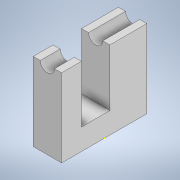
# Autodesk Inventor part: shaft_support
Saved by Autodesk Inventor 2021 (Build 250183000, 183)
## iProperties
Created: 2021-04-13
Part Number: shaft_support
Material: Generic
Document SubType Name: Modeling
Designer: Jawal
Density: 1 g/cm^3
Appearance: Default
Author: Jawal
Autodesk Inventor part; units mm, degrees
note: some values were not read from the file. Chosen so that the rebuilt part matches the saved one: direction of "Emboss1".
ref_plane "YZ Plane" through (0, 0, 0) normal (1, 0, 0) x (0, 1, 0)
ref_plane "XZ Plane" through (0, 0, 0) normal (0, 1, 0) x (-1, 0, 0)
ref_plane "XY Plane" through (0, 0, 0) normal (0, 0, 1) x (1, 0, 0)
sketch "Sketch1" plane through (0, 0, 0) normal (0, 1, 0) x (-1, 0, 0)
  line L0 (5, 15) -> (-5, 15)
  line L1 (-5, 15) -> (-5, -15)
  line L2 (-5, -15) -> (5, -15)
  line L3 (5, -15) -> (5, 15)
  point P0 (0, 0)
  dimension "d0" = 30
  dimension "d1" = 10
  dimension "d2" = 5
  dimension "d3" = 15
  constraints: 8 end point, 2 parallel, 1 horizontal, 1 perpendicular
  measures "d0" distance of L2.end L0.start
  measures "d1" distance of L1.end L2.end
  measures "d2" distance from line of L3 point (0, 0)
  measures "d3" distance from line of point (0, 0) L0
extrude "Extrusion1" add sketch "Sketch1" along normal blind 27.5
sketch "Sketch4" plane through (5, 0, 15) normal (1, 0, 0) x (0, 0, -1)
  point P0 (15, 0)
sketch "Sketch5" plane through (5, 0, 15) normal (1, 0, 0) x (0, 0, -1)
  line L0 (7, 27.5) -> (17, 27.5)
  line L1 (17, 27.5) -> (17, 7.5)
  line L2 (17, 7.5) -> (7, 7.5)
  line L3 (7, 7.5) -> (7, 27.5)
  line L4 (0, 0) -> (0, 27.5) projected
  line L5 (30, 0) -> (30, 27.5) projected
  point P0 (15, 0)
  dimension "d12" = 7
  dimension "d14" = 10
  dimension "d15" = 20
  constraints: 8 end point, 2 parallel, 1 horizontal, 1 perpendicular
  measures "d12" distance between parallel lines of L4 L3
  measures "d14" distance of L0.start L0.end
  measures "d15" distance of L0.end L1.end
extrude "Extrusion4" cut sketch "Sketch5" against normal through all
sketch "Sketch6" plane through (-5, 0, 15) normal (0, 0, 1) x (1, 0, 0)
  line L0 (10, 27.5) -> (0, 27.5) projected
  arc A0 (2.5, 27.5) -> (7.5, 27.5) centre (5, 27.5) ccw
  line L1 (2.5, 27.5) -> (7.5, 27.5)
  point P0 (5, 0)
  dimension "d18" = 5
  constraints: 2 end point, 2 point on circle, 2 point on line, 1 centre point, 1 collinear, 1 midpoint
  measures "d18" diameter of A0
extrude "Extrusion5" cut sketch "Sketch6" against normal through all
sketch "Sketch8" plane through (0, 0, 0) normal (0, -1, 0) x (1, 0, 0)
  circle A0 centre (0, -4) radius 1.5
  line L0 (5, -15) -> (-5, -15) projected
  line L1 (-5, 15) -> (5, 15) projected
  point P0 (0, 0)
  dimension "d24" = 3
  dimension "d28" = 19
  constraints: 1 centre point
  measures "d24" diameter of A0
  measures "d28" distance from line of L1 A0.centre
extrude "Extrusion6" add sketch "Sketch8" along normal blind 3
sketch "Sketch9" plane through (-5, 0, -15) normal (-1, 0, 0) x (0, 0, 1)
  line L0 (9.262, 5.0823) -> (36.8865, 5.0823) construction
  line L1 (36.8865, 5.0823) -> (36.8865, -0.8197) construction
  line L2 (36.8865, -0.8197) -> (9.262, -0.8197) construction
  line L3 (9.262, -0.8197) -> (9.262, 5.0823) construction
  spline S0 degree 2 poles (10.0221, 3.0109) (9.8049, 3.0109) (9.5002, 3.1017) (9.3657, 3.1665) knots 0 0 0 1 2 2 2
  line L4 (9.3657, 3.1665) -> (9.3657, 3.5004)
  line L5 (9.3657, 3.5004) -> (9.3851, 3.5004)
  spline S1 degree 2 poles (9.3851, 3.5004) (9.5164, 3.3772) (9.8487, 3.2411) (10.0027, 3.2411) knots 0 0 0 1 2 2 2
  spline S2 degree 2 poles (10.0027, 3.2411) (10.2231, 3.2411) (10.4484, 3.4242) (10.4484, 3.575) knots 0 0 0 1 2 2 2
  spline S3 degree 2 poles (10.4484, 3.575) (10.4484, 3.6949) (10.33, 3.844) (10.202, 3.8813) knots 0 0 0 1 2 2 2
  spline S4 degree 2 poles (10.202, 3.8813) (10.1096, 3.9072) (9.9557, 3.9429) (9.8406, 3.972) knots 0 0 0 1 2 2 2
  spline S5 degree 2 poles (9.8406, 3.972) (9.7369, 3.9996) (9.5732, 4.0823) (9.5099, 4.1487) knots 0 0 0 1 2 2 2
  spline S6 degree 2 poles (9.5099, 4.1487) (9.4484, 4.2152) (9.3803, 4.3934) (9.3803, 4.5101) knots 0 0 0 1 2 2 2
  spline S7 degree 2 poles (9.3803, 4.5101) (9.3803, 4.7532) (9.7595, 5.0823) (10.0529, 5.0823) knots 0 0 0 1 2 2 2
  spline S8 degree 2 poles (10.0529, 5.0823) (10.2215, 5.0823) (10.5197, 5.0158) (10.6477, 4.9526) knots 0 0 0 1 2 2 2
  line L6 (10.6477, 4.9526) -> (10.6477, 4.6349)
  line L7 (10.6477, 4.6349) -> (10.6283, 4.6349)
  spline S9 degree 2 poles (10.6283, 4.6349) (10.5326, 4.7224) (10.2344, 4.8521) (10.0707, 4.8521) knots 0 0 0 1 2 2 2
  spline S10 degree 2 poles (10.0707, 4.8521) (9.886, 4.8521) (9.6574, 4.6787) (9.6574, 4.5377) knots 0 0 0 1 2 2 2
  spline S11 degree 2 poles (9.6574, 4.5377) (9.6574, 4.4113) (9.792, 4.2605) (9.9184, 4.2265) knots 0 0 0 1 2 2 2
  spline S12 degree 2 poles (9.9184, 4.2265) (10.0027, 4.2038) (10.2474, 4.1455) (10.3284, 4.1211) knots 0 0 0 1 2 2 2
  spline S13 degree 2 poles (10.3284, 4.1211) (10.5343, 4.0579) (10.7255, 3.8035) (10.7255, 3.6171) knots 0 0 0 1 2 2 2
  spline S14 degree 2 poles (10.7255, 3.6171) (10.7255, 3.4988) (10.6299, 3.2719) (10.544, 3.1925) knots 0 0 0 1 2 2 2
  spline S15 degree 2 poles (10.544, 3.1925) (10.4484, 3.1049) (10.2052, 3.0109) (10.0221, 3.0109) knots 0 0 0 1 2 2 2
  line L8 (12.1437, 3.0466) -> (11.8908, 3.0466)
  line L9 (11.8908, 3.0466) -> (11.8908, 3.2119)
  spline S16 degree 2 poles (11.8908, 3.2119) (11.7741, 3.1098) (11.5651, 3.0045) (11.4354, 3.0045) knots 0 0 0 1 2 2 2
  spline S17 degree 2 poles (11.4354, 3.0045) (11.3381, 3.0045) (11.1647, 3.0693) (11.1015, 3.139) knots 0 0 0 1 2 2 2
  spline S18 degree 2 poles (11.1015, 3.139) (11.0367, 3.2087) (10.9654, 3.421) (10.9654, 3.5733) knots 0 0 0 1 2 2 2
  line L10 (10.9654, 3.5733) -> (10.9654, 4.5474)
  line L11 (10.9654, 4.5474) -> (11.2182, 4.5474)
  line L12 (11.2182, 4.5474) -> (11.2182, 3.6917)
  spline S19 degree 2 poles (11.2182, 3.6917) (11.2182, 3.5717) (11.236, 3.4145) (11.2668, 3.3562) knots 0 0 0 1 2 2 2
  spline S20 degree 2 poles (11.2668, 3.3562) (11.2976, 3.2978) (11.403, 3.2443) (11.5018, 3.2443) knots 0 0 0 1 2 2 2
  spline S21 degree 2 poles (11.5018, 3.2443) (11.5942, 3.2443) (11.8033, 3.3497) (11.8908, 3.4258) knots 0 0 0 1 2 2 2
  line L13 (11.8908, 3.4258) -> (11.8908, 4.5474)
  line L14 (11.8908, 4.5474) -> (12.1437, 4.5474)
  line L15 (12.1437, 4.5474) -> (12.1437, 3.0466)
  spline S22 degree 2 poles (13.7676, 3.8375) (13.7676, 3.4615) (13.4095, 3.0174) (13.1356, 3.0174) knots 0 0 0 1 2 2 2
  spline S23 degree 2 poles (13.1356, 3.0174) (13.0237, 3.0174) (12.8519, 3.0693) (12.7628, 3.1228) knots 0 0 0 1 2 2 2
  line L16 (12.7628, 3.1228) -> (12.7628, 2.4939)
  line L17 (12.7628, 2.4939) -> (12.5099, 2.4939)
  line L18 (12.5099, 2.4939) -> (12.5099, 4.5474)
  line L19 (12.5099, 4.5474) -> (12.7628, 4.5474)
  line L20 (12.7628, 4.5474) -> (12.7628, 4.3902)
  spline S24 degree 2 poles (12.7628, 4.3902) (12.8568, 4.4761) (13.0869, 4.5895) (13.2215, 4.5895) knots 0 0 0 1 2 2 2
  spline S25 degree 2 poles (13.2215, 4.5895) (13.4792, 4.5895) (13.7676, 4.1811) (13.7676, 3.8375) knots 0 0 0 1 2 2 2
  spline S26 degree 2 poles (13.5067, 3.8083) (13.5067, 4.066) (13.343, 4.3497) (13.1599, 4.3497) knots 0 0 0 1 2 2 2
  spline S27 degree 2 poles (13.1599, 4.3497) (13.0529, 4.3497) (12.8519, 4.2541) (12.7628, 4.1795) knots 0 0 0 1 2 2 2
  line L21 (12.7628, 4.1795) -> (12.7628, 3.327)
  spline S28 degree 2 poles (12.7628, 3.327) (12.8616, 3.28) (13.0027, 3.2443) (13.0934, 3.2443) knots 0 0 0 1 2 2 2
  spline S29 degree 2 poles (13.0934, 3.2443) (13.2895, 3.2443) (13.5067, 3.5328) (13.5067, 3.8083) knots 0 0 0 1 2 2 2
  spline S30 degree 2 poles (15.2879, 3.8375) (15.2879, 3.4615) (14.9297, 3.0174) (14.6558, 3.0174) knots 0 0 0 1 2 2 2
  spline S31 degree 2 poles (14.6558, 3.0174) (14.544, 3.0174) (14.3722, 3.0693) (14.283, 3.1228) knots 0 0 0 1 2 2 2
  line L22 (14.283, 3.1228) -> (14.283, 2.4939)
  line L23 (14.283, 2.4939) -> (14.0302, 2.4939)
  line L24 (14.0302, 2.4939) -> (14.0302, 4.5474)
  line L25 (14.0302, 4.5474) -> (14.283, 4.5474)
  line L26 (14.283, 4.5474) -> (14.283, 4.3902)
  spline S32 degree 2 poles (14.283, 4.3902) (14.377, 4.4761) (14.6072, 4.5895) (14.7417, 4.5895) knots 0 0 0 1 2 2 2
  spline S33 degree 2 poles (14.7417, 4.5895) (14.9994, 4.5895) (15.2879, 4.1811) (15.2879, 3.8375) knots 0 0 0 1 2 2 2
  spline S34 degree 2 poles (15.027, 3.8083) (15.027, 4.066) (14.8633, 4.3497) (14.6801, 4.3497) knots 0 0 0 1 2 2 2
  spline S35 degree 2 poles (14.6801, 4.3497) (14.5732, 4.3497) (14.3722, 4.2541) (14.283, 4.1795) knots 0 0 0 1 2 2 2
  line L27 (14.283, 4.1795) -> (14.283, 3.327)
  spline S36 degree 2 poles (14.283, 3.327) (14.3819, 3.28) (14.5229, 3.2443) (14.6137, 3.2443) knots 0 0 0 1 2 2 2
  spline S37 degree 2 poles (14.6137, 3.2443) (14.8098, 3.2443) (15.027, 3.5328) (15.027, 3.8083) knots 0 0 0 1 2 2 2
  spline S38 degree 2 poles (16.7839, 3.797) (16.7839, 3.4177) (16.4192, 3.0045) (16.1145, 3.0045) knots 0 0 0 1 2 2 2
  spline S39 degree 2 poles (16.1145, 3.0045) (15.8017, 3.0045) (15.4435, 3.4307) (15.4435, 3.797) knots 0 0 0 1 2 2 2
  spline S40 degree 2 poles (15.4435, 3.797) (15.4435, 4.173) (15.813, 4.5895) (16.1145, 4.5895) knots 0 0 0 1 2 2 2
  spline S41 degree 2 poles (16.1145, 4.5895) (16.4192, 4.5895) (16.7839, 4.1746) (16.7839, 3.797) knots 0 0 0 1 2 2 2
  spline S42 degree 2 poles (16.5229, 3.797) (16.5229, 4.0887) (16.3106, 4.3724) (16.1145, 4.3724) knots 0 0 0 1 2 2 2
  spline S43 degree 2 poles (16.1145, 4.3724) (15.9184, 4.3724) (15.7044, 4.0887) (15.7044, 3.797) knots 0 0 0 1 2 2 2
  spline S44 degree 2 poles (15.7044, 3.797) (15.7044, 3.5134) (15.9184, 3.2216) (16.1145, 3.2216) knots 0 0 0 1 2 2 2
  spline S45 degree 2 poles (16.1145, 3.2216) (16.309, 3.2216) (16.5229, 3.5085) (16.5229, 3.797) knots 0 0 0 1 2 2 2
  line L28 (17.839, 4.2767) -> (17.826, 4.2767)
  spline S46 degree 2 poles (17.826, 4.2767) (17.7968, 4.2848) (17.7336, 4.2881) (17.6899, 4.2881) knots 0 0 0 1 2 2 2
  spline S47 degree 2 poles (17.6899, 4.2881) (17.5877, 4.2881) (17.3868, 4.1989) (17.296, 4.1114) knots 0 0 0 1 2 2 2
  line L29 (17.296, 4.1114) -> (17.296, 3.0466)
  line L30 (17.296, 3.0466) -> (17.0432, 3.0466)
  line L31 (17.0432, 3.0466) -> (17.0432, 4.5474)
  line L32 (17.0432, 4.5474) -> (17.296, 4.5474)
  line L33 (17.296, 4.5474) -> (17.296, 4.3237)
  spline S48 degree 2 poles (17.296, 4.3237) (17.4338, 4.4469) (17.6396, 4.5474) (17.7369, 4.5474) knots 0 0 0 1 2 2 2
  spline S49 degree 2 poles (17.7369, 4.5474) (17.7757, 4.5474) (17.8146, 4.5442) (17.839, 4.5393) knots 0 0 0 1 2 2 2
  line L34 (17.839, 4.5393) -> (17.839, 4.2767)
  spline S50 degree 2 poles (18.4889, 3.0174) (18.283, 3.0174) (18.0513, 3.2524) (18.0513, 3.5069) knots 0 0 0 1 2 2 2
  line L35 (18.0513, 3.5069) -> (18.0513, 4.3383)
  line L36 (18.0513, 4.3383) -> (17.8811, 4.3383)
  line L37 (17.8811, 4.3383) -> (17.8811, 4.5474)
  line L38 (17.8811, 4.5474) -> (18.0513, 4.5474)
  line L39 (18.0513, 4.5474) -> (18.0513, 4.9785)
  line L40 (18.0513, 4.9785) -> (18.3041, 4.9785)
  line L41 (18.3041, 4.9785) -> (18.3041, 4.5474)
  line L42 (18.3041, 4.5474) -> (18.7693, 4.5474)
  line L43 (18.7693, 4.5474) -> (18.7693, 4.3383)
  line L44 (18.7693, 4.3383) -> (18.3041, 4.3383)
  line L45 (18.3041, 4.3383) -> (18.3041, 3.6236)
  spline S51 degree 2 poles (18.3041, 3.6236) (18.3041, 3.5101) (18.3122, 3.3853) (18.3398, 3.3318) knots 0 0 0 1 2 2 2
  spline S52 degree 2 poles (18.3398, 3.3318) (18.3625, 3.2848) (18.4646, 3.2378) (18.5521, 3.2378) knots 0 0 0 1 2 2 2
  spline S53 degree 2 poles (18.5521, 3.2378) (18.6137, 3.2378) (18.7287, 3.2751) (18.7547, 3.2865) knots 0 0 0 1 2 2 2
  line L46 (18.7547, 3.2865) -> (18.7693, 3.2865)
  line L47 (18.7693, 3.2865) -> (18.7693, 3.0596)
  spline S54 degree 2 poles (18.7693, 3.0596) (18.698, 3.0401) (18.5521, 3.0174) (18.4889, 3.0174) knots 0 0 0 1 2 2 2
  line L48 (19.6185, 3.0466) -> (20.2928, 5.0466)
  line L49 (20.2928, 5.0466) -> (20.6202, 5.0466)
  line L50 (20.6202, 5.0466) -> (21.2944, 3.0466)
  line L51 (21.2944, 3.0466) -> (21.014, 3.0466)
  line L52 (21.014, 3.0466) -> (20.8325, 3.6058)
  line L53 (20.8325, 3.6058) -> (20.0691, 3.6058)
  line L54 (20.0691, 3.6058) -> (19.8876, 3.0466)
  line L55 (19.8876, 3.0466) -> (19.6185, 3.0466)
  line L56 (20.7595, 3.8327) -> (20.45, 4.7743)
  line L57 (20.45, 4.7743) -> (20.142, 3.8327)
  line L58 (20.142, 3.8327) -> (20.7595, 3.8327)
  point P0 (15, 0)
  constraints: 2 other
emboss "Emboss1" sketch "Sketch9" operation cut depth 1 direction (1, 0, 0)
equation "\"d2\" = 0.5 * d1"
equation "\"d3\" = 0.5 * d0"
body "Solid1"
